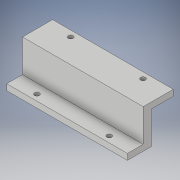
# Autodesk Inventor part: EBoardStandoffs
Saved by Autodesk Inventor 2019 (Build 230136000, 136)
## iProperties
Created: 2018-12-23
Part Number: EBoardStandoffs
Material: Generic
Document SubType Name: Modeling
Designer: james
Density: 1 g/cm^3
Appearance: Default
Author: james
Autodesk Inventor part; units mm, degrees
ref_plane "YZ Plane" through (0, 0, 0) normal (1, 0, 0) x (0, 1, 0)
ref_plane "XZ Plane" through (0, 0, 0) normal (0, 1, 0) x (-1, 0, 0)
ref_plane "XY Plane" through (0, 0, 0) normal (0, 0, 1) x (1, 0, 0)
sketch "Sketch1" plane through (0, 0, 0) normal (0, 1, 0) x (-1, 0, 0)
  line L0 (11.4626, 9.6064) -> (-115.5374, 9.6064)
  line L1 (-115.5374, 9.6064) -> (-115.5374, -15.7936)
  line L2 (-115.5374, -15.7936) -> (11.4626, -15.7936)
  line L3 (11.4626, -15.7936) -> (11.4626, 9.6064)
  point P0 (0, 0)
  dimension "d0" = 25.4
  dimension "d1" = 127
  constraints: 8 end point, 2 parallel, 1 horizontal, 1 perpendicular
  measures "d0" distance of L2.end L0.start
  measures "d1" distance of L0.start L0.end
extrude "Extrusion1" add sketch "Sketch1" along normal blind 6.35
sketch "Sketch2" plane through (0, 6.35, 0) normal (0, 1, 0) x (1, 0, 0)
  line L0 (115.5374, 15.7936) -> (-11.4626, 15.7936) projected
  line L1 (-11.4626, 15.7936) -> (-11.4626, -9.6064) projected
  line L2 (115.5374, -9.6064) -> (115.5374, 15.7936) projected
  line L3 (-11.4626, 15.7936) -> (115.5374, 15.7936)
  line L4 (115.5374, 15.7936) -> (115.5374, 3.0936)
  line L5 (115.5374, 3.0936) -> (-11.4626, 3.0936)
  line L6 (-11.4626, 3.0936) -> (-11.4626, 15.7936)
  point P0 (0, 0)
  dimension "d31" = 12.7
  constraints: 8 end point, 2 parallel, 1 horizontal, 1 midpoint, 1 perpendicular
  measures "d31" distance between parallel lines of L0 L5
extrude "Extrusion2" add sketch "Sketch2" along normal blind 27.94
sketch "Sketch3" plane through (0, 34.29, 0) normal (0, 1, 0) x (1, 0, 0)
  line L0 (-11.4626, 3.0936) -> (115.5374, 3.0936) projected
  line L1 (-11.4626, 15.7936) -> (-11.4626, 3.0936) projected
  line L2 (115.5374, 15.7936) -> (-11.4626, 15.7936) projected
  line L3 (115.5374, 3.0936) -> (115.5374, 15.7936) projected
  line L4 (-11.4626, 3.0936) -> (115.5374, 3.0936)
  line L5 (115.5374, 3.0936) -> (115.5374, 38.6536)
  line L6 (115.5374, 38.6536) -> (-11.4626, 38.6536)
  line L7 (-11.4626, 38.6536) -> (-11.4626, 3.0936)
  point P0 (0, 0)
  dimension "d6" = 35.56
  constraints: 8 end point, 2 parallel, 1 horizontal, 1 perpendicular
  measures "d6" distance between parallel lines of L0 L6
extrude "Extrusion3" add sketch "Sketch3" along normal blind 6.35
sketch "Sketch4" plane through (0, 40.64, 0) normal (0, 1, 0) x (1, 0, 0)
  line L0 (115.5374, 38.6536) -> (-11.4626, 38.6536) projected
  line L1 (-11.4626, 38.6536) -> (-11.4626, 3.0936) projected
  point P0 (0, 0)
  point P1 (13.9374, 32.3036)
  point P2 (90.1374, 32.3036)
  dimension "d9" = 0
  dimension "d10" = 6.35
  dimension "d11" = 76.2
  dimension "d12" = 25.4
  measures "d9" vertical distance of point (90.137, 32.304) point (13.937, 32.304)
  measures "d10" distance from line of L0 point (13.937, 32.304)
  measures "d11" distance of point (90.137, 32.304) point (13.937, 32.304)
  measures "d12" distance from line of L1 point (13.937, 32.304)
hole "Hole1" at (13.9374, 40.64, -32.3036) at (90.1374, 40.64, -32.3036) direction (0, -1, 0) diameter 5.08 end through all
sketch "Sketch5" plane through (0, 6.35, 0) normal (0, 1, 0) x (1, 0, 0)
  line L0 (-11.4626, -9.6064) -> (115.5374, -9.6064) projected
  line L1 (115.5374, -9.6064) -> (115.5374, 3.0936) projected
  point P0 (0, 0)
  point P1 (13.9374, -3.2564)
  point P2 (90.1374, -3.2564)
  dimension "d20" = 0
  dimension "d21" = 6.35
  dimension "d22" = 25.4
  dimension "d23" = 76.2
  measures "d20" vertical distance of point (13.937, -3.256) point (90.137, -3.256)
  measures "d21" distance from line of L0 point (90.137, -3.256)
  measures "d22" distance from line of L1 point (90.137, -3.256)
  measures "d23" distance of point (90.137, -3.256) point (13.937, -3.256)
hole "Hole2" at (13.9374, 6.35, 3.2564) at (90.1374, 6.35, 3.2564) direction (0, -1, 0) diameter 5.08 end through all
sketch "Sketch7" plane through (0, 40.64, 0) normal (0, 1, 0) x (1, 0, 0)
  line L0 (-11.4626, 3.0936) -> (115.5374, 3.0936) projected
  line L1 (-11.4626, 38.6536) -> (-11.4626, 3.0936) projected
  line L2 (115.5374, 3.0936) -> (115.5374, 38.6536) projected
  line L3 (-11.4626, 3.0936) -> (115.5374, 3.0936)
  line L4 (115.5374, 3.0936) -> (115.5374, 7.0306)
  line L5 (115.5374, 7.0306) -> (-11.4626, 7.0306)
  line L6 (-11.4626, 7.0306) -> (-11.4626, 3.0936)
  point P0 (0, 0)
  dimension "d35" = 3.937
  constraints: 8 end point, 2 parallel, 1 horizontal, 1 perpendicular, 1 point on line
  measures "d35" distance between parallel lines of L0 L5
extrude "Extrusion5" cut sketch "Sketch7" against normal blind 34.29
body "Solid1"
